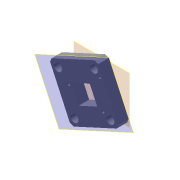
# Autodesk Inventor part: 10_Adapter_KES400_Thorlabs
Saved by Autodesk Inventor 2019 (Build 230136000, 136)
## iProperties
Created: 2019-05-03
Part Number: 10_Adapter_KES400_Thorlabs
Material: Generic
Document SubType Name: Modeling
Designer: diederichbenedict
Density: 1 g/cm^3
Appearance: Default
Author: diederichbenedict
Autodesk Inventor part; units mm, degrees
ref_plane "YZ Plane" through (0, 0, 0) normal (1, 0, 0) x (0, 1, 0)
ref_plane "XZ Plane" through (0, 0, 0) normal (0, 1, 0) x (-1, 0, 0)
ref_plane "XY Plane" through (0, 0, 0) normal (0, 0, 1) x (1, 0, 0)
ref_plane "Work Plane1" through (0, 0, 0) normal (0, 0, 1) x (1, 0, 0)
ref_plane "Work Plane2" through (13.4154, -42.9082, 9) normal (0, 0, -1) x (-0.9086751, -0.417504, 0)
sketch "Sketch1" plane through (13.4154, -42.9082, 9) normal (0, 0, -1) x (-0.9086751, -0.417504, 0)
  line L0 (20.066, 26.9166) -> (20.066, 62.7742) projected
  line L1 (20.066, 62.7742) -> (17.9288, 64.9114) projected
  line L2 (17.9288, 64.9114) -> (-17.9288, 64.9114) projected
  line L3 (-17.9288, 64.9114) -> (-20.066, 62.7742) projected
  line L4 (-20.066, 62.7742) -> (-20.066, 26.9166) projected
  line L5 (-20.066, 26.9166) -> (-17.9288, 24.7794) projected
  line L6 (-17.9288, 24.7794) -> (17.9288, 24.7794) projected
  line L7 (17.9288, 24.7794) -> (20.066, 26.9166) projected
  circle A0 centre (-15, 59.8454) radius 3.2639 projected
  circle A1 centre (15, 59.8454) radius 3.2639 projected
  circle A2 centre (-15, 29.8455) radius 3.2639 projected
  circle A3 centre (15, 29.8455) radius 3.2639 projected
  circle A4 centre (0, 44.8454) radius 13.3985 projected
  line L8 (8, 50.8454) -> (-7.5, 50.8454) construction
  line L9 (-7.5, 50.8454) -> (-7.5, 37.3454) construction
  line L10 (-7.5, 37.3454) -> (8, 37.3454) construction
  line L11 (8, 37.3454) -> (8, 50.8454) construction
  circle A5 centre (-17.5, 54.8454) radius 1 construction
  circle A6 centre (-11, 34.3454) radius 1 construction
  circle A7 centre (10.5, 49.8454) radius 1 construction
  arc A8 (-15.8555, 56.5454) -> (-16.8555, 57.5454) centre (-16.8555, 56.5454) ccw construction
  line L12 (-15.8555, 56.5454) -> (-15.8555, 53.8078) construction
  arc A9 (-15.8555, 53.8078) -> (-14.8555, 52.8078) centre (-14.8555, 53.8078) ccw construction
  line L13 (-14.8555, 52.8078) -> (12, 52.8078) construction
  arc A10 (13, 51.8078) -> (12, 52.8078) centre (12, 51.8078) ccw construction
  line L14 (13, 51.8078) -> (13, 49.2425) construction
  arc A11 (12, 48.2425) -> (13, 49.2425) centre (12, 49.2425) ccw construction
  line L15 (12, 48.2425) -> (11, 48.2425) construction
  arc A12 (11, 48.2425) -> (10, 47.2425) centre (11, 47.2425) ccw construction
  line L16 (10, 47.2425) -> (10, 35.7078) construction
  line L17 (10, 35.7078) -> (-8.4723, 35.7078) construction
  arc A13 (-8.4723, 35.7078) -> (-9.4723, 34.7078) centre (-8.4723, 34.7078) ccw construction
  line L18 (-9.4723, 34.7078) -> (-9.4723, 32.8454) construction
  arc A14 (-10.4723, 31.8454) -> (-9.4723, 32.8454) centre (-10.4723, 32.8454) ccw construction
  line L19 (-10.4723, 31.8454) -> (-20, 31.8454) construction
  line L20 (-20, 31.8454) -> (-20, 57.5454) construction
  line L21 (-20, 57.5454) -> (-16.8555, 57.5454) construction
  line L22 (8, 37.3454) -> (-7.5, 37.3454)
  line L23 (-7.5, 37.3454) -> (-7.5, 50.8454)
  line L24 (-7.5, 50.8454) -> (8, 50.8454)
  line L25 (8, 50.8454) -> (8, 37.3454)
  circle A15 centre (10.5, 49.8454) radius 1
  circle A16 centre (-17.5, 54.8454) radius 1
  circle A17 centre (-11, 34.3454) radius 1
  circle A18 centre (15, 29.8455) radius 3.05
  circle A19 centre (-15, 29.8455) radius 3.05
  circle A20 centre (-15, 59.8454) radius 3.05
  circle A21 centre (15, 59.8454) radius 3.05
  point P0 (-5.7241, 44.5906)
  dimension "d2" = 6.1
  dimension "d3" = 6.1
  dimension "d4" = 6.1
  dimension "d5" = 6.1
  constraints: 8 end point, 7 centre point, 7 coincident, 3 concentric, 2 parallel, 1 horizontal, 1 perpendicular
  measures "d2" diameter of A18
  measures "d3" diameter of A19
  measures "d4" diameter of A20
  measures "d5" diameter of A21
extrude "Extrusion1" add sketch "Sketch1" along normal blind 8 contours L7 L6 L5 L4 L3 L2 L1 L0 | A0 | A1 | A2 | A3 | A4
body "Solid1"
